Autodesk Fusion 360 part; units mm, degrees
(part 2 of 2)
sketch "Sketch17" plane through (0, 0, -2) normal (0, 0, -1) x (1, 0, 0)
  line L0 (194.147805, 28.451903) -> (190.147805, 28.451903)
  line L1 (190.147805, 28.451903) -> (190.147805, 68.451903)
  line L2 (190.147805, 68.451903) -> (194.147805, 68.451903)
  line L3 (194.147805, 68.451903) -> (194.147805, 28.451903)
  line L4 (190.147805, 135.548097) -> (190.147805, 175.548097)
  line L5 (190.147805, 175.548097) -> (194.147805, 175.548097)
  line L6 (194.147805, 175.548097) -> (194.147805, 135.548097)
  line L7 (194.147805, 135.548097) -> (190.147805, 135.548097)
  circle A0 centre (13.149146, 10.944513) radius 2.5
  arc A1 (71.144783, 62.444513) -> (73.644783, 59.944735) centre (71.144783, 59.944513) ccw
  line L8 (71.144783, 62.444513) -> (13.147805, 62.444513)
  circle A2 centre (13.149146, 59.944513) radius 2.5
  line L9 (13.147805, 62.444513) -> (13.147805, 178)
  line L10 (13.147805, 178) -> (179.147805, 178)
  line L11 (179.147805, 178) -> (179.147805, 26)
  line L12 (179.147805, 26) -> (73.647801, 26)
  line L13 (73.647801, 26) -> (73.644783, 59.944735)
  line L14 (205.147805, 26.032876) -> (205.147805, 177.967124)
  line L15 (205.147805, 177.967124) -> (371.147805, 177.967124)
  line L16 (371.147805, 177.967124) -> (371.147805, 26.032876)
  line L17 (371.147805, 26.032876) -> (205.147805, 26.032876)
  arc A3 (380.935047, 102.943024) -> (384.47223, 101.075414) centre (382.708118, 102.017702) ccw
  arc A4 (384.47223, 101.075414) -> (380.935047, 102.943024) centre (382.69916, 102.000736) ccw
  arc A5 (198.107947, 103.961473) -> (198.34915, 99.968762) centre (198.233029, 101.965388) ccw
  arc A6 (198.34915, 99.968762) -> (198.107947, 103.961473) centre (198.224067, 101.964847) ccw
  circle A7 centre (186.071543, 101.964847) radius 2
  circle A8 centre (1.596451, 102.000736) radius 2
  circle A9 centre (96.149998, 192.999996) radius 2
  circle A10 centre (96.147805, 10.951903) radius 2
  line L18 (388.743999, 209.096194) -> (-4.448389, 209.096194)
  arc A11 (-4.448389, 209.096194) -> (-10.930518, 202.114535) centre (-4.448389, 202.596194) ccw
  line L19 (-10.930518, 202.114535) -> (-10.939432, 102)
  line L20 (-10.939432, 102) -> (-10.930518, 1.885465)
  arc A12 (-10.930518, 1.885465) -> (-4.448389, -5.096194) centre (-4.448389, 1.403806) ccw
  line L21 (-4.448389, -5.096194) -> (388.743999, -5.096194)
  arc A13 (388.743999, -5.096194) -> (395.243999, 1.403816) centre (388.743999, 1.403806) ccw
  line L22 (395.243999, 1.403806) -> (395.243999, 202.596194)
  arc A14 (395.243999, 202.596194) -> (388.743999, 209.096194) centre (388.743999, 202.596194) ccw
  arc A15 (286.156007, 193.203633) -> (290.136075, 192.804906) centre (288.146469, 193.008543) ccw
  arc A16 (290.136075, 192.804906) -> (286.156007, 193.203633) centre (288.145613, 192.999996) ccw
  arc A17 (287.260608, 12.744354) -> (289.052067, 9.168) centre (288.16487, 10.960451) ccw
  arc A18 (289.052067, 9.168) -> (287.260608, 12.744354) centre (288.147805, 10.951903) ccw
  circle A19 centre (71.149146, 10.944513) radius 2.5
  circle A20 centre (-4.448389, 202.596194) radius 5.5
  circle A21 centre (388.743999, 202.596194) radius 5.5
  circle A22 centre (388.743999, 1.403806) radius 5.5
  circle A23 centre (-4.448389, 1.403806) radius 5.5
  line L23 (-9.948389, 1.403806) -> (-9.948389, 202.596194)
  line L24 (-4.448389, 208.096194) -> (388.743999, 208.096194)
  line L25 (394.243999, 202.596194) -> (394.243999, 1.403806)
  line L26 (388.743999, -4.096194) -> (-4.448389, -4.096194)
  dimension "d213" = 11
  dimension "d214" = 11
  dimension "d215" = 11
  dimension "d216" = 11
  constraint concentric A11 A20
  constraint concentric A14 A21
  constraint concentric A13 A22
  constraint concentric A12 A23
  constraint tangent A20 L23
  constraint vertical L23
  constraint tangent A21 L24
  constraint perpendicular L23 L24
  constraint tangent A22 L25
  constraint perpendicular L24 L25
  constraint tangent A23 L26
  constraint perpendicular L25 L26
  measures "d213" diameter of A20
  measures "d214" diameter of A21
  measures "d215" diameter of A22
  measures "d216" diameter of A23
extrude "Extrude22" add sketch "Sketch17" along normal blind 25 contours L18 A11 L19 L20 A12 L21 A13 L22 A14 picked at (126.615741, 208.429527) bodies 5
sketch "Sketch18" plane through (-10.930351, 0.000973, 0) normal (-1, 0.00008904, 0) x (-0.00008904, -1, 0)
  line L0 (102.000974, 0) -> (1.886438, 0)
  line L1 (1.886438, 0) -> (1.886438, -27)
  line L2 (1.886438, -27) -> (102.000974, -27)
  line L3 (102.000974, -27) -> (102.000974, 0)
  circle A0 centre (4.636438, -27) radius 2.75
  dimension "d219" = 5.5
  measures "d219" diameter of A0
extrude "Extrude23" cut sketch "Sketch18" against normal blind 2 contours L2 A0 picked at (5.51238, -26.729808) bodies 5
sketch "Sketch19" plane through (0, 0, -27) normal (0, 0, -1) x (1, 0, 0)
  line L0 (-10.931008, 7.385465) -> (-9.948389, 7.385552)
  line L1 (-9.948389, 7.385552) -> (-9.948389, 202.596194)
  arc A0 (-4.448389, 208.096194) -> (-9.948389, 202.596194) centre (-4.448389, 202.596194) ccw
  line L2 (-4.448389, 208.096194) -> (388.743999, 208.096194)
  arc A1 (394.243999, 202.596194) -> (388.743999, 208.096194) centre (388.743999, 202.596194) ccw
  line L3 (394.243999, 202.596194) -> (394.243999, 1.403806)
  arc A2 (388.743999, -4.096194) -> (394.243999, 1.403806) centre (388.743999, 1.403806) ccw
  line L4 (388.743999, -4.096194) -> (-4.448389, -4.096194)
  arc A3 (-9.948389, 1.403806) -> (-4.448389, -4.096194) centre (-4.448389, 1.403806) ccw
  line L5 (-9.948389, 1.403806) -> (-9.948389, 1.885552)
  line L6 (-9.948389, 1.885552) -> (-10.930518, 1.885465)
  arc A4 (-10.930518, 1.885465) -> (-4.448389, -5.096194) centre (-4.448389, 1.403806) ccw
  line L7 (-4.448389, -5.096194) -> (388.743999, -5.096194)
  arc A5 (388.743999, -5.096194) -> (395.243999, 1.403806) centre (388.743999, 1.403806) ccw
  line L8 (395.243999, 1.403806) -> (395.243999, 202.596194)
  arc A6 (395.243999, 202.596194) -> (388.743999, 209.096194) centre (388.743999, 202.596194) ccw
  line L9 (388.743999, 209.096194) -> (-4.448389, 209.096194)
  arc A7 (-4.448389, 209.096194) -> (-10.930518, 202.114535) centre (-4.448389, 202.596194) ccw
  line L10 (-10.930518, 202.114535) -> (-10.939432, 102)
  line L11 (-10.939432, 102) -> (-10.931008, 7.385465)
  circle A8 centre (-4.448389, 202.596194) radius 6.5
  circle A9 centre (-4.448389, 1.403806) radius 6.5
  circle A10 centre (388.743999, 1.403806) radius 6.5
  circle A11 centre (388.743999, 202.596194) radius 6.5
  line L12 (388.743999, 209.096194) -> (-4.448389, 209.096194)
  line L13 (-10.947379, 202.710792) -> (-10.946884, 1.263926)
  line L14 (-4.448389, -5.096194) -> (388.743999, -5.096194)
  line L15 (395.243999, 1.403806) -> (395.243999, 202.596194)
  constraint concentric A0 A8
  constraint concentric A3 A9
  constraint concentric A2 A10
  constraint concentric A1 A11
  constraint tangent A8 L12
  constraint tangent A10 L14
  constraint tangent A11 L15
extrude "Extrude24" add sketch "Sketch19" along normal blind 2 separate body contours L0 L1 L10 L11 A8 | L0 L1 L2 L3 L4 A4 A7 L10 L11 A8 A9 A10 A11 L13 | L1 A0 L2 A7 A8 L13 | L1 A0 L2 A8 | L2 L9 A8 A11 L12 | A4 A9 L13 | L4 A3 L5 L6 A4 A9 L13 | L2 A1 L3 A6 A11 | L2 A1 L3 A11 | L4 A3 L5 L6 A9 | L3 L8 A10 A11 L15 | L4 L7 A9 A10 L14 | L3 A2 L4 A5 A10 | L3 A2 L4 A10 picked at (-10.278737, 102.839215) picked at (255.811015, 69.387281) picked at (-10.568787, 203.237986) picked at (-4.647868, 203.006515) picked at (127.770441, 208.383498) picked at (-10.94733, 1.388248) picked at (-10.567397, 0.746022) picked at (389.313259, 208.722147) picked at (389.045268, 202.897463) picked at (-4.667667, 1.176486) picked at (394.531304, 69.622636) picked at (256.525169, -4.383498) picked at (394.869952, 0.834547) picked at (389.045268, 1.102537) makes body 6
sketch "Sketch20" plane through (0, 0, -27) normal (0, 0, 1) x (-1, 0, 0)
  line L0 (-395.243999, 202.596194) -> (-395.243999, 1.403806)
  arc A0 (-395.243999, 1.403806) -> (-388.743999, -5.096194) centre (-388.743999, 1.403806) ccw
  line L1 (-388.743999, -5.096194) -> (4.448389, -5.096194)
  arc A1 (4.448389, -5.096194) -> (10.946884, 1.543654) centre (4.448389, 1.403806) ccw
  line L2 (10.946884, 1.543654) -> (10.947379, 202.710792)
  arc A2 (10.947379, 202.710792) -> (4.448389, 209.096194) centre (4.448389, 202.596194) ccw
  line L3 (4.448389, 209.096194) -> (-388.743999, 209.096194)
  arc A3 (-388.743999, 209.096194) -> (-395.243999, 202.596194) centre (-388.743999, 202.596194) ccw
  circle A4 centre (-388.743999, 1.403806) radius 5.5
  circle A5 centre (-388.743999, 1.403806) radius 4.5
  line L4 (-388.743999, 1.403806) -> (-388.743999, -4.096194)
  line L5 (-388.743999, 1.403806) -> (-394.243999, 1.403806)
  circle A6 centre (-388.743999, 202.596194) radius 5.5
  circle A7 centre (-388.743999, 202.596194) radius 4.5
  line L6 (-388.743999, 202.596194) -> (-388.743999, 208.096194)
  line L7 (-388.743999, 202.596194) -> (-394.243999, 202.596194)
  circle A8 centre (4.448389, 202.596194) radius 5.5
  circle A9 centre (4.448389, 202.596194) radius 4.5
  line L8 (4.448389, 202.596194) -> (9.948389, 202.596194)
  line L9 (4.448389, 202.596194) -> (4.448389, 208.096194)
  circle A10 centre (4.448389, 1.403806) radius 5.5
  circle A11 centre (4.448389, 1.403806) radius 4.5
  line L10 (4.448389, 1.403806) -> (4.448389, -4.096194)
  line L11 (4.448389, 1.403806) -> (9.948389, 1.403806)
  line L12 (4.448389, -4.096194) -> (-388.743999, -4.096194) construction
  line L13 (4.448389, 208.096194) -> (-388.743999, 208.096194) construction
  line L14 (-192.147805, 208.096194) -> (-192.147805, -4.096194) construction
  line L15 (-192.147805, -4.096194) -> (-190.147805, -4.096194) construction
  line L16 (-192.147805, -4.096194) -> (-194.147805, -4.096194) construction
  line L17 (-190.147805, -4.096194) -> (-175.147805, -4.096194)
  line L18 (-175.147805, -4.096194) -> (-175.147805, -2.096194)
  line L19 (-175.147805, -2.096194) -> (-190.147805, -2.096194)
  line L20 (-190.147805, -2.096194) -> (-190.147805, -4.096194)
  line L21 (-194.147805, -4.096194) -> (-209.147805, -4.096194)
  line L22 (-209.147805, -4.096194) -> (-209.147805, -2.096194)
  line L23 (-209.147805, -2.096194) -> (-194.147805, -2.096194)
  line L24 (-194.147805, -2.096194) -> (-194.147805, -4.096194)
  line L25 (-192.147805, 102) -> (-395.243999, 102) construction
  line L26 (-192.147805, 102) -> (10.947131, 102.127223) construction
  line L27 (-175.147805, 206.096194) -> (-190.147805, 206.096194)
  line L28 (-175.147805, 208.096194) -> (-175.147805, 206.096194)
  line L29 (-190.147805, 208.096194) -> (-175.147805, 208.096194)
  line L30 (-190.147805, 206.096194) -> (-190.147805, 208.096194)
  line L31 (-194.147805, 206.096194) -> (-194.147805, 208.096194)
  line L32 (-209.147805, 206.096194) -> (-194.147805, 206.096194)
  line L33 (-194.147805, 208.096194) -> (-209.147805, 208.096194)
  line L34 (-209.147805, 208.096194) -> (-209.147805, 206.096194)
  dimension "d224" = 11
  dimension "d225" = 9
  dimension "d226" = 11
  dimension "d227" = 9
  dimension "d228" = 11
  dimension "d229" = 9
  dimension "d230" = 11
  dimension "d231" = 9
  dimension "d232" = 2
  dimension "d233" = 2
  dimension "d234" = 15
  dimension "d235" = 2
  dimension "d236" = 15
  dimension "d237" = 2
  constraint concentric A0 A4
  constraint concentric A0 A5
  constraint perpendicular L1 L4
  constraint perpendicular L4 L5
  constraint concentric A3 A6
  constraint concentric A6 A7
  constraint vertical L6
  constraint perpendicular L6 L7
  constraint concentric A2 A8
  constraint concentric A8 A9
  constraint horizontal L8
  constraint perpendicular L8 L9
  constraint concentric A1 A10
  constraint concentric A1 A11
  constraint vertical L10
  constraint perpendicular L10 L11
  constraint perpendicular L14 L15
  constraint perpendicular L14 L16
  constraint horizontal L17
  constraint vertical L18
  constraint horizontal L19
  constraint vertical L20
  constraint horizontal L21
  constraint vertical L22
  constraint horizontal L23
  constraint vertical L24
  measures "d224" diameter of A4
  measures "d225" diameter of A5
  measures "d226" diameter of A6
  measures "d227" diameter of A7
  measures "d228" diameter of A8
  measures "d229" diameter of A9
  measures "d230" diameter of A10
  measures "d231" diameter of A11
extrude "Extrude25" add sketch "Sketch20" along normal blind 10 contours A4 A5 L4 L5 | A5 L4 L5 | A6 A7 L6 L7 | A7 L6 L7 | A8 A9 L8 L9 | A9 L8 L9 | A10 A11 L10 L11 | A11 L10 L11 | L17 L18 L19 L20 | L21 L22 L23 L24 | L27 L28 L29 L30 | L31 L32 L33 L34 picked at (-393.876737, 0.929423) picked at (-391.728731, 1.190334) picked at (-393.892005, 202.857105) picked at (-390.859915, 204.71211) picked at (6.149092, 207.462163) picked at (6.241641, 204.991699) picked at (4.709299, -3.7442) picked at (7.433121, 1.190334) picked at (-185.147805, -2.762861) picked at (-199.147805, -3.429527) picked at (-180.147805, 207.429527) picked at (-199.147805, 207.429527) bodies 6
split "Split4" by plane through (192.152272, -102.254102, 6.25) normal (-1, 0.00004452, 0) bodies 6 5 makes body 8 at (34.022313, -32.296184, 0) makes body 7 at (124.452561, -68.514551, -29)
sketch "Sketch21" plane through (-10.930351, 0.000973, 0) normal (-1, 0.00008904, 0) x (-0.00008904, -1, 0)
  arc A0 (7.386438, -27) -> (1.886438, -27) centre (4.636438, -27) ccw
  line L0 (7.386438, -27) -> (102.000974, -27)
  line L1 (102.000974, -27) -> (102.000974, 0)
  line L2 (102.000974, 0) -> (1.886438, 0)
  line L3 (1.886438, 0) -> (1.886438, -27)
  line L4 (102.000974, 0) -> (102.000974, -27) construction
  line L5 (112.000974, -6.75) -> (92.000974, -6.75)
  line L6 (92.000974, -6.75) -> (92.000974, -20.25)
  line L7 (92.000974, -20.25) -> (112.000974, -20.25)
  line L8 (112.000974, -20.25) -> (112.000974, -6.75)
  line L9 (112.000974, -6.75) -> (92.000974, -20.25) construction
  line L10 (92.000974, -6.75) -> (112.000974, -20.25) construction
  point P0 (102.000974, -13.5)
  dimension "d240" = 20
  dimension "d241" = 13.5
  constraint horizontal L5
  constraint perpendicular L5 L6
  constraint parallel L5 L7
  constraint parallel L6 L8
extrude "Extrude26" cut sketch "Sketch21" against normal blind 2 contours L1 L5 L6 L7 | L1 L5 L7 L8 picked at (98.66764, -15.75) picked at (105.334307, -11.25) bodies 8
equation "d16 = ( 192 * 2 ) * 1 mm"
equation "d87 = ( 192 * 2 ) * 1 mm"
equation "d139 = ( 192 * 2 ) * 1 mm"
